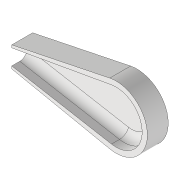
# Autodesk Inventor part: Weiche_1
Saved by Autodesk Inventor 2020 (Build 240168000, 168)
## iProperties
Created: 2020-04-19
Part Number: Weiche_1
Material: Generisch
Document SubType Name: Modeling
Designer: franz
Density: 1 g/cm^3
Appearance: Vorgabe
Author: franz
Autodesk Inventor part; units mm, degrees
ref_plane "YZ Plane" through (0, 0, 0) normal (1, 0, 0) x (0, 1, 0)
ref_plane "XZ Plane" through (0, 0, 0) normal (0, 1, 0) x (-1, 0, 0)
ref_plane "XY Plane" through (0, 0, 0) normal (0, 0, 1) x (1, 0, 0)
sketch "Skizze1" plane through (0, 0, 0) normal (0, 0, 1) x (1, 0, 0)
  arc A0 (-4.018, -29.7297) -> (-4.018, 29.7297) centre (0, 0) ccw
  line L0 (-4.018, 29.7297) -> (-150, 10)
  line L1 (-150, 10) -> (-150, -10)
  line L2 (-150, -10) -> (-4.018, -29.7297)
  line L3 (-186, 0) -> (66, 0) projected
  dimension "d0" = 60
  dimension "d1" = 150
  dimension "d2" = 20
  constraints: 6 end point, 2 point on circle, 2 tangent, 1 centre point, 1 coincident, 1 vertical, 1 other
  measures "d0" diameter of A0
  measures "d1" distance from line of point (0, 0) L1
  measures "d2" distance of L0.end L1.end
extrude "Extrusion1" add sketch "Skizze1" along normal blind 40
sketch "Skizze2" plane through (0, 0, 40) normal (0, 0, 1) x (1, 0, 0)
  line L0 (-150, 10) -> (-150, -10) projected
  line L1 (-150, 7.5) -> (-2.9253, 24.8283)
  arc A0 (-2.9253, -24.8283) -> (-2.9253, 24.8283) centre (0, 0) ccw
  line L2 (-150, -7.5) -> (-2.9253, -24.8283)
  line L3 (-186, 0) -> (66, 0) projected
  dimension "d5" = 15
  dimension "d6" = 25
  constraints: 4 end point, 2 point on circle, 2 point on line, 2 tangent, 1 centre point, 1 coincident, 1 other
  measures "d5" distance of L2.start L1.start
  measures "d6" radius of A0
extrude "Extrusion2" cut sketch "Skizze2" against normal blind 35
fillet "Rundung1" radius 7.3 3 edges at (25, 0, 5) (-76.4626, -16.1641, 5) (-76.4626, 16.1641, 5)
